Autodesk Inventor part; units mm, degrees
(part 2 of 3)
  measures "d19" distance of L6.end L4.start
  measures "d20" distance between parallel lines of L1 L7
  measures "d21" distance of L0.start L1.end
  measures "d22" distance between parallel lines of L0 L4
extrude "Extrusion4" cut sketch "Sketch4" against normal blind 5.08 contours S0 L8 L9 S1 S2 S3 S4 S5 S6 S7 S8 L10 L11 S9 S10 S11 S12 S13 S14 S15 | S16 S17 L12 L13 L14 S18 S19 S20 S21 L15 L16 L17 S22 S23 | S24 S25 L18 L19 L20 S26 S27 S28 L21 S29 | L28 L29 L30 L31 | S38 S39 L32 L33 L34 S40 S41 S42 L35 S43 | L42 L43 L44 L45 L46 L47 L48 L49 | S52 L53 L54 S53 S54 S55 S56 S57 S58 S59 S60 L55 L56 S61 S62 S63 S64 S65 S66 S67 | L57 L58 L59 L60 L61 L62 L63 L64 L65 L66 L67 L68 | L69 L70 L71 L72 L73 L74 L75 L76 L77 L78 | S68 S69 S70 S71 S72 S73 S74 S75 | S82 S83 L79 L80 L81 S84 S85 S86 S87 L82 L83 L84 S88 S89 | L85 L86 L87 L88 L89 L90 L91 S90 S91 S92 L92 | L96 L97 L98 L99 L100 L101 L102 L103 L104 L105 L106 L107 | L108 L109 L110 L111 L112 L113 L114 L115 L116 L117 L118 L119 | L120 L121 L122 L123 L124 L125 L126 S97 S98 S99 L127 | L131 L132 L133 L134 L135 L136 L137 L138 | L139 L150 L146 | L146 L150 L151 L152 L153 L154 L155 L156 L157 | L139 L140 L141 L142 L143 L144 L145 S104 S105 S106 L146 L150 | L161 L162 L163 L164 L165 L166 L167 L168 L169 L170 | S111 L171 L172 S112 S113 S114 S115 S116 S117 S118 S119 L173 L174 S120 S121 S122 S123 S124 S125 S126 | L175 L176 L177 L178 L179 L180 L181 L182 L183 L184 | S127 S128 S129 S130 S131 S132 S133 S134 | L185 L186 L187 L188 L189 L190 L191 S141 S142 S143 L192 | L196 L197 L198 L199 L200 L201 L202 L203 L204 L205 L206 L207 L208
sketch "Sketch5" plane through (0, -25.4, 0) normal (0, -1, 0) x (1, 0, 0)
  line L0 (0, 0) -> (203.2, 0) projected
  line L1 (203.2, 50.8) -> (0, 50.8) projected
  line L2 (0, 50.8) -> (0, 0) projected
  line L3 (203.2, 0) -> (203.2, 50.8) projected
  line L4 (8.4667, 48.26) -> (110.0667, 48.26) construction
  line L5 (110.0667, 48.26) -> (110.0667, 2.54) construction
  line L6 (110.0667, 2.54) -> (8.4667, 2.54) construction
  line L7 (8.4667, 2.54) -> (8.4667, 48.26) construction
  line L8 (118.5333, 38.1) -> (194.7333, 38.1) construction
  line L9 (194.7333, 38.1) -> (194.7333, 12.7) construction
  line L10 (194.7333, 12.7) -> (118.5333, 12.7) construction
  line L11 (118.5333, 12.7) -> (118.5333, 38.1) construction
  spline S0 degree 2 poles (23.465, 39.4772) (23.465, 38.2768) (21.9978, 36.9726) (20.7603, 36.9726) knots 0 0 0 1 2 2 2
  spline S1 degree 2 poles (20.7603, 36.9726) (20.4639, 36.9726) (19.4784, 37.0764) (19.145, 37.1505) knots 0 0 0 1 2 2 2
  line L12 (19.145, 37.1505) -> (19.145, 38.3213)
  line L13 (19.145, 38.3213) -> (19.2116, 38.3213)
  spline S2 degree 2 poles (19.2116, 38.3213) (19.4636, 38.2323) (20.212, 38.0249) (20.5973, 38.0249) knots 0 0 0 1 2 2 2
  spline S3 degree 2 poles (20.5973, 38.0249) (21.1605, 38.0249) (21.8348, 38.2842) (21.9904, 38.5213) knots 0 0 0 1 2 2 2
  spline S4 degree 2 poles (21.9904, 38.5213) (22.1608, 38.7659) (22.2498, 39.4772) (22.2498, 39.9441) knots 0 0 0 1 2 2 2
  line L14 (22.2498, 39.9441) -> (22.2498, 45.2719)
  line L15 (22.2498, 45.2719) -> (20.3157, 45.2719)
  line L16 (20.3157, 45.2719) -> (20.3157, 46.2426)
  line L17 (20.3157, 46.2426) -> (23.465, 46.2426)
  line L18 (23.465, 46.2426) -> (23.465, 39.4772)
  spline S5 degree 2 poles (28.452, 36.9059) (27.6443, 36.9059) (26.4439, 37.3283) (26.0215, 37.7507) knots 0 0 0 1 2 2 2
  spline S6 degree 2 poles (26.0215, 37.7507) (25.5398, 38.2249) (25.1471, 39.5587) (25.1471, 40.5369) knots 0 0 0 1 2 2 2
  line L19 (25.1471, 40.5369) -> (25.1471, 46.2426)
  line L20 (25.1471, 46.2426) -> (26.3623, 46.2426)
  line L21 (26.3623, 46.2426) -> (26.3623, 40.5369)
  spline S7 degree 2 poles (26.3623, 40.5369) (26.3623, 39.8996) (26.5254, 39.04) (26.7551, 38.6918) knots 0 0 0 1 2 2 2
  spline S8 degree 2 poles (26.7551, 38.6918) (26.9996, 38.3213) (27.8444, 37.9433) (28.452, 37.9433) knots 0 0 0 1 2 2 2
  spline S9 degree 2 poles (28.452, 37.9433) (29.0226, 37.9433) (29.9118, 38.3213) (30.1563, 38.6918) knots 0 0 0 1 2 2 2
  spline S10 degree 2 poles (30.1563, 38.6918) (30.386, 39.04) (30.549, 39.8922) (30.549, 40.5072) knots 0 0 0 1 2 2 2
  line L22 (30.549, 40.5072) -> (30.549, 46.2426)
  line L23 (30.549, 46.2426) -> (31.7643, 46.2426)
  line L24 (31.7643, 46.2426) -> (31.7643, 40.5369)
  spline S11 degree 2 poles (31.7643, 40.5369) (31.7643, 39.581) (31.3789, 38.2175) (30.8899, 37.7507) knots 0 0 0 1 2 2 2
  spline S12 degree 2 poles (30.8899, 37.7507) (30.4527, 37.3209) (29.2967, 36.9059) (28.452, 36.9059) knots 0 0 0 1 2 2 2
  spline S13 degree 2 poles (36.0547, 36.9356) (35.0617, 36.9356) (33.6687, 37.3505) (33.0536, 37.6469) knots 0 0 0 1 2 2 2
  line L25 (33.0536, 37.6469) -> (33.0536, 39.1734)
  line L26 (33.0536, 39.1734) -> (33.1425, 39.1734)
  spline S14 degree 2 poles (33.1425, 39.1734) (33.7428, 38.6103) (35.2618, 37.9878) (35.9658, 37.9878) knots 0 0 0 1 2 2 2
  spline S15 degree 2 poles (35.9658, 37.9878) (36.9735, 37.9878) (38.0035, 38.8251) (38.0035, 39.5143) knots 0 0 0 1 2 2 2
  spline S16 degree 2 poles (38.0035, 39.5143) (38.0035, 40.0626) (37.4626, 40.7443) (36.8772, 40.9148) knots 0 0 0 1 2 2 2
  spline S17 degree 2 poles (36.8772, 40.9148) (36.4548, 41.0333) (35.7509, 41.1964) (35.2248, 41.3297) knots 0 0 0 1 2 2 2
  spline S18 degree 2 poles (35.2248, 41.3297) (34.7505, 41.4557) (34.0021, 41.8336) (33.7131, 42.1374) knots 0 0 0 1 2 2 2
  spline S19 degree 2 poles (33.7131, 42.1374) (33.4315, 42.4412) (33.1203, 43.2564) (33.1203, 43.7899) knots 0 0 0 1 2 2 2
  spline S20 degree 2 poles (33.1203, 43.7899) (33.1203, 44.9014) (34.8543, 46.4056) (36.1955, 46.4056) knots 0 0 0 1 2 2 2
  spline S21 degree 2 poles (36.1955, 46.4056) (36.9661, 46.4056) (38.3296, 46.1018) (38.915, 45.8128) knots 0 0 0 1 2 2 2
  line L27 (38.915, 45.8128) -> (38.915, 44.3605)
  line L28 (38.915, 44.3605) -> (38.826, 44.3605)
  spline S22 degree 2 poles (38.826, 44.3605) (38.3889, 44.7606) (37.0254, 45.3534) (36.277, 45.3534) knots 0 0 0 1 2 2 2
  spline S23 degree 2 poles (36.277, 45.3534) (35.4322, 45.3534) (34.3874, 44.5605) (34.3874, 43.9158) knots 0 0 0 1 2 2 2
  spline S24 degree 2 poles (34.3874, 43.9158) (34.3874, 43.3379) (35.0025, 42.6487) (35.5804, 42.4931) knots 0 0 0 1 2 2 2
  spline S25 degree 2 poles (35.5804, 42.4931) (35.9658, 42.3894) (37.0847, 42.1226) (37.4552, 42.0115) knots 0 0 0 1 2 2 2
  spline S26 degree 2 poles (37.4552, 42.0115) (38.3963, 41.7225) (39.2706, 40.5591) (39.2706, 39.7069) knots 0 0 0 1 2 2 2
  spline S27 degree 2 poles (39.2706, 39.7069) (39.2706, 39.166) (38.8335, 38.1286) (38.4407, 37.7655) knots 0 0 0 1 2 2 2
  spline S28 degree 2 poles (38.4407, 37.7655) (38.0035, 37.3654) (36.892, 36.9356) (36.0547, 36.9356) knots 0 0 0 1 2 2 2
  line L29 (42.6422, 37.0986) -> (42.6422, 45.1607)
  line L30 (42.6422, 45.1607) -> (39.5745, 45.1607)
  line L31 (39.5745, 45.1607) -> (39.5745, 46.2426)
  line L32 (39.5745, 46.2426) -> (46.9252, 46.2426)
  line L33 (46.9252, 46.2426) -> (46.9252, 45.1607)
  line L34 (46.9252, 45.1607) -> (43.8575, 45.1607)
  line L35 (43.8575, 45.1607) -> (43.8575, 37.0986)
  line L36 (43.8575, 37.0986) -> (42.6422, 37.0986)
  line L37 (51.0378, 37.0986) -> (47.4958, 37.0986)
  line L38 (47.4958, 37.0986) -> (47.4958, 38.0323)
  line L39 (47.4958, 38.0323) -> (48.6592, 38.0323)
  line L40 (48.6592, 38.0323) -> (48.6592, 45.3089)
  line L41 (48.6592, 45.3089) -> (47.4958, 45.3089)
  line L42 (47.4958, 45.3089) -> (47.4958, 46.2426)
  line L43 (47.4958, 46.2426) -> (51.0378, 46.2426)
  line L44 (51.0378, 46.2426) -> (51.0378, 45.3089)
  line L45 (51.0378, 45.3089) -> (49.8744, 45.3089)
  line L46 (49.8744, 45.3089) -> (49.8744, 38.0323)
  line L47 (49.8744, 38.0323) -> (51.0378, 38.0323)
  line L48 (51.0378, 38.0323) -> (51.0378, 37.0986)
  line L49 (59.0851, 37.0986) -> (57.7217, 37.0986)
  line L50 (57.7217, 37.0986) -> (53.6758, 44.9829)
  line L51 (53.6758, 44.9829) -> (53.6758, 37.0986)
  line L52 (53.6758, 37.0986) -> (52.542, 37.0986)
  line L53 (52.542, 37.0986) -> (52.542, 46.2426)
  line L54 (52.542, 46.2426) -> (54.2686, 46.2426)
  line L55 (54.2686, 46.2426) -> (57.9514, 39.003)
  line L56 (57.9514, 39.003) -> (57.9514, 46.2426)
  line L57 (57.9514, 46.2426) -> (59.0851, 46.2426)
  line L58 (59.0851, 46.2426) -> (59.0851, 37.0986)
  line L59 (63.8794, 37.0986) -> (66.962, 46.2426)
  line L60 (66.962, 46.2426) -> (68.4588, 46.2426)
  line L61 (68.4588, 46.2426) -> (71.5414, 37.0986)
  line L62 (71.5414, 37.0986) -> (70.2595, 37.0986)
  line L63 (70.2595, 37.0986) -> (69.4295, 39.6551)
  line L64 (69.4295, 39.6551) -> (65.9394, 39.6551)
  line L65 (65.9394, 39.6551) -> (65.1095, 37.0986)
  line L66 (65.1095, 37.0986) -> (63.8794, 37.0986)
  line L67 (69.0961, 40.6925) -> (67.6808, 44.9977)
  line L68 (67.6808, 44.9977) -> (66.2729, 40.6925)
  line L69 (66.2729, 40.6925) -> (69.0961, 40.6925)
  line L70 (77.7066, 37.0986) -> (72.4084, 37.0986)
  line L71 (72.4084, 37.0986) -> (72.4084, 46.2426)
  line L72 (72.4084, 46.2426) -> (73.6236, 46.2426)
  line L73 (73.6236, 46.2426) -> (73.6236, 38.1805)
  line L74 (73.6236, 38.1805) -> (77.7066, 38.1805)
  line L75 (77.7066, 38.1805) -> (77.7066, 37.0986)
  line L76 (83.9607, 37.0986) -> (78.6625, 37.0986)
  line L77 (78.6625, 37.0986) -> (78.6625, 46.2426)
  line L78 (78.6625, 46.2426) -> (79.8777, 46.2426)
  line L79 (79.8777, 46.2426) -> (79.8777, 38.1805)
  line L80 (79.8777, 38.1805) -> (83.9607, 38.1805)
  line L81 (83.9607, 38.1805) -> (83.9607, 37.0986)
  line L82 (84.9165, 37.0986) -> (84.9165, 46.2426)
  line L83 (84.9165, 46.2426) -> (90.6371, 46.2426)
  line L84 (90.6371, 46.2426) -> (90.6371, 45.1607)
  line L85 (90.6371, 45.1607) -> (86.1318, 45.1607)
  line L86 (86.1318, 45.1607) -> (86.1318, 42.6561)
  line L87 (86.1318, 42.6561) -> (90.3333, 42.6561)
  line L88 (90.3333, 42.6561) -> (90.3333, 41.5743)
  line L89 (90.3333, 41.5743) -> (86.1318, 41.5743)
  line L90 (86.1318, 41.5743) -> (86.1318, 38.1805)
  line L91 (86.1318, 38.1805) -> (90.6371, 38.1805)
  line L92 (90.6371, 38.1805) -> (90.6371, 37.0986)
  line L93 (90.6371, 37.0986) -> (84.9165, 37.0986)
  line L94 (98.514, 37.0986) -> (97.1505, 37.0986)
  line L95 (97.1505, 37.0986) -> (93.1047, 44.9829)
  line L96 (93.1047, 44.9829) -> (93.1047, 37.0986)
  line L97 (93.1047, 37.0986) -> (91.9709, 37.0986)
  line L98 (91.9709, 37.0986) -> (91.9709, 46.2426)
  line L99 (91.9709, 46.2426) -> (93.6975, 46.2426)
  line L100 (93.6975, 46.2426) -> (97.3802, 39.003)
  line L101 (97.3802, 39.003) -> (97.3802, 46.2426)
  line L102 (97.3802, 46.2426) -> (98.514, 46.2426)
  line L103 (98.514, 46.2426) -> (98.514, 37.0986)
  line L104 (27.9889, 22.0432) -> (31.0714, 31.1872)
  line L105 (31.0714, 31.1872) -> (32.5683, 31.1872)
  line L106 (32.5683, 31.1872) -> (35.6508, 22.0432)
  line L107 (35.6508, 22.0432) -> (34.3689, 22.0432)
  line L108 (34.3689, 22.0432) -> (33.539, 24.5997)
  line L109 (33.539, 24.5997) -> (30.0488, 24.5997)
  line L110 (30.0488, 24.5997) -> (29.2189, 22.0432)
  line L111 (29.2189, 22.0432) -> (27.9889, 22.0432)
  line L112 (33.2055, 25.6371) -> (31.7902, 29.9424)
  line L113 (31.7902, 29.9424) -> (30.3823, 25.6371)
  line L114 (30.3823, 25.6371) -> (33.2055, 25.6371)
  line L115 (41.4381, 22.0432) -> (36.9772, 22.0432)
  line L116 (36.9772, 22.0432) -> (36.9772, 22.9769)
  line L117 (36.9772, 22.9769) -> (38.6371, 22.9769)
  line L118 (38.6371, 22.9769) -> (38.6371, 29.105)
  line L119 (38.6371, 29.105) -> (36.9772, 29.105)
  line L120 (36.9772, 29.105) -> (36.9772, 29.9424)
  spline S29 degree 2 poles (36.9772, 29.9424) (37.9183, 29.9424) (38.8075, 30.4759) (38.8668, 31.2169) knots 0 0 0 1 2 2 2
  line L121 (38.8668, 31.2169) -> (39.8153, 31.2169)
  line L122 (39.8153, 31.2169) -> (39.8153, 22.9769)
  line L123 (39.8153, 22.9769) -> (41.4381, 22.9769)
  line L124 (41.4381, 22.9769) -> (41.4381, 22.0432)
  line L125 (49.0037, 25.1851) -> (47.9145, 25.1851)
  line L126 (47.9145, 25.1851) -> (47.9145, 22.0432)
  line L127 (47.9145, 22.0432) -> (46.7363, 22.0432)
  line L128 (46.7363, 22.0432) -> (46.7363, 25.1851)
  line L129 (46.7363, 25.1851) -> (42.6978, 25.1851)
  line L130 (42.6978, 25.1851) -> (42.6978, 26.4745)
  line L131 (42.6978, 26.4745) -> (46.7881, 31.1872)
  line L132 (46.7881, 31.1872) -> (47.9145, 31.1872)
  line L133 (47.9145, 31.1872) -> (47.9145, 26.1706)
  line L134 (47.9145, 26.1706) -> (49.0037, 26.1706)
  line L135 (49.0037, 26.1706) -> (49.0037, 25.1851)
  line L136 (46.7363, 26.1706) -> (46.7363, 29.7423)
  line L137 (46.7363, 29.7423) -> (43.6611, 26.1706)
  line L138 (43.6611, 26.1706) -> (46.7363, 26.1706)
  spline S30 degree 2 poles (55.5246, 24.948) (55.5246, 24.2885) (55.1022, 23.1622) (54.7169, 22.7472) knots 0 0 0 1 2 2 2
  spline S31 degree 2 poles (54.7169, 22.7472) (54.3316, 22.3322) (53.183, 21.8506) (52.4717, 21.8506) knots 0 0 0 1 2 2 2
  spline S32 degree 2 poles (52.4717, 21.8506) (51.8196, 21.8506) (50.545, 22.1396) (50.0782, 22.3693) knots 0 0 0 1 2 2 2
  line L139 (50.0782, 22.3693) -> (50.0782, 23.666)
  line L140 (50.0782, 23.666) -> (50.1671, 23.666)
  spline S33 degree 2 poles (50.1671, 23.666) (50.3079, 23.5623) (50.834, 23.2955) (51.1527, 23.177) knots 0 0 0 1 2 2 2
  spline S34 degree 2 poles (51.1527, 23.177) (51.5158, 23.051) (52.116, 22.9102) (52.4939, 22.9102) knots 0 0 0 1 2 2 2
  spline S35 degree 2 poles (52.4939, 22.9102) (52.8644, 22.9102) (53.5609, 23.177) (53.8129, 23.466) knots 0 0 0 1 2 2 2
  spline S36 degree 2 poles (53.8129, 23.466) (54.0426, 23.7401) (54.2797, 24.4663) (54.2797, 24.9554) knots 0 0 0 1 2 2 2
  spline S37 degree 2 poles (54.2797, 24.9554) (54.2797, 25.4445) (54.0129, 26.0669) (53.761, 26.2744) knots 0 0 0 1 2 2 2
  spline S38 degree 2 poles (53.761, 26.2744) (53.5016, 26.5041) (52.731, 26.6968) (52.2642, 26.6968) knots 0 0 0 1 2 2 2
  spline S39 degree 2 poles (52.2642, 26.6968) (51.7603, 26.6968) (50.7599, 26.5411) (50.4561, 26.4745) knots 0 0 0 1 2 2 2
  line L141 (50.4561, 26.4745) -> (50.4561, 31.1872)
  line L142 (50.4561, 31.1872) -> (55.4727, 31.1872)
  line L143 (55.4727, 31.1872) -> (55.4727, 30.1128)
  line L144 (55.4727, 30.1128) -> (51.6343, 30.1128)
  line L145 (51.6343, 30.1128) -> (51.6343, 27.6749)
  spline S40 degree 2 poles (51.6343, 27.6749) (51.8566, 27.7045) (52.2864, 27.7268) (52.4642, 27.7268) knots 0 0 0 1 2 2 2
  spline S41 degree 2 poles (52.4642, 27.7268) (53.1682, 27.7268) (54.1389, 27.497) (54.5835, 27.1562) knots 0 0 0 1 2 2 2
  spline S42 degree 2 poles (54.5835, 27.1562) (55.0355, 26.8153) (55.5246, 25.7779) (55.5246, 24.948) knots 0 0 0 1 2 2 2
  spline S43 degree 2 poles (62.6234, 25.0073) (62.6234, 24.3033) (62.1566, 23.1103) (61.7639, 22.7102) knots 0 0 0 1 2 2 2
  spline S44 degree 2 poles (61.7639, 22.7102) (61.3563, 22.2878) (60.3337, 21.8506) (59.7187, 21.8506) knots 0 0 0 1 2 2 2
  spline S45 degree 2 poles (59.7187, 21.8506) (59.1036, 21.8506) (58.0885, 22.2655) (57.7031, 22.6805) knots 0 0 0 1 2 2 2
  spline S46 degree 2 poles (57.7031, 22.6805) (57.2289, 23.177) (56.6954, 24.8442) (56.6954, 26.0595) knots 0 0 0 1 2 2 2
  spline S47 degree 2 poles (56.6954, 26.0595) (56.6954, 27.2525) (57.1844, 29.1717) (57.6957, 29.8831) knots 0 0 0 1 2 2 2
  spline S48 degree 2 poles (57.6957, 29.8831) (58.1922, 30.5796) (59.7631, 31.3577) (60.7931, 31.3577) knots 0 0 0 1 2 2 2
  spline S49 degree 2 poles (60.7931, 31.3577) (61.0969, 31.3577) (61.6305, 31.2984) (61.8305, 31.2317) knots 0 0 0 1 2 2 2
  line L146 (61.8305, 31.2317) -> (61.8305, 30.0535)
  line L147 (61.8305, 30.0535) -> (61.7787, 30.0535)
  spline S50 degree 2 poles (61.7787, 30.0535) (61.6082, 30.1424) (60.9858, 30.298) (60.6301, 30.298) knots 0 0 0 1 2 2 2
  spline S51 degree 2 poles (60.6301, 30.298) (59.489, 30.298) (58.0885, 28.7568) (57.9551, 27.2451) knots 0 0 0 1 2 2 2
  spline S52 degree 2 poles (57.9551, 27.2451) (58.3923, 27.5489) (59.3111, 27.8824) (59.8595, 27.8824) knots 0 0 0 1 2 2 2
  spline S53 degree 2 poles (59.8595, 27.8824) (60.393, 27.8824) (61.1933, 27.6675) (61.6305, 27.3414) knots 0 0 0 1 2 2 2
  spline S54 degree 2 poles (61.6305, 27.3414) (62.1344, 26.9635) (62.6234, 25.7927) (62.6234, 25.0073) knots 0 0 0 1 2 2 2
  spline S55 degree 2 poles (61.3785, 24.9554) (61.3785, 25.5186) (61.0821, 26.2818) (60.7561, 26.5486) knots 0 0 0 1 2 2 2
  spline S56 degree 2 poles (60.7561, 26.5486) (60.5116, 26.7412) (59.9039, 26.8672) (59.5853, 26.8672) knots 0 0 0 1 2 2 2
  spline S57 degree 2 poles (59.5853, 26.8672) (59.1555, 26.8672) (58.3478, 26.6078) (57.9551, 26.3633) knots 0 0 0 1 2 2 2
  spline S58 degree 2 poles (57.9551, 26.3633) (57.9477, 26.2299) (57.9329, 25.978) (57.9329, 25.7853) knots 0 0 0 1 2 2 2
  spline S59 degree 2 poles (57.9329, 25.7853) (57.9329, 24.8368) (58.3034, 23.6735) (58.5849, 23.3696) knots 0 0 0 1 2 2 2
  spline S60 degree 2 poles (58.5849, 23.3696) (58.8443, 23.0807) (59.4075, 22.8509) (59.7261, 22.8509) knots 0 0 0 1 2 2 2
  spline S61 degree 2 poles (59.7261, 22.8509) (60.4671, 22.8509) (61.3785, 23.9032) (61.3785, 24.9554) knots 0 0 0 1 2 2 2
  spline S62 degree 2 poles (69.4851, 25.0073) (69.4851, 24.3033) (69.0183, 23.1103) (68.6256, 22.7102) knots 0 0 0 1 2 2 2
  spline S63 degree 2 poles (68.6256, 22.7102) (68.218, 22.2878) (67.1954, 21.8506) (66.5804, 21.8506) knots 0 0 0 1 2 2 2
  spline S64 degree 2 poles (66.5804, 21.8506) (65.9654, 21.8506) (64.9502, 22.2655) (64.5649, 22.6805) knots 0 0 0 1 2 2 2
  spline S65 degree 2 poles (64.5649, 22.6805) (64.0906, 23.177) (63.5571, 24.8442) (63.5571, 26.0595) knots 0 0 0 1 2 2 2
  spline S66 degree 2 poles (63.5571, 26.0595) (63.5571, 27.2525) (64.0461, 29.1717) (64.5574, 29.8831) knots 0 0 0 1 2 2 2
  spline S67 degree 2 poles (64.5574, 29.8831) (65.0539, 30.5796) (66.6248, 31.3577) (67.6548, 31.3577) knots 0 0 0 1 2 2 2
  spline S68 degree 2 poles (67.6548, 31.3577) (67.9587, 31.3577) (68.4922, 31.2984) (68.6922, 31.2317) knots 0 0 0 1 2 2 2
  line L148 (68.6922, 31.2317) -> (68.6922, 30.0535)
  line L149 (68.6922, 30.0535) -> (68.6404, 30.0535)
  spline S69 degree 2 poles (68.6404, 30.0535) (68.4699, 30.1424) (67.8475, 30.298) (67.4918, 30.298) knots 0 0 0 1 2 2 2
  spline S70 degree 2 poles (67.4918, 30.298) (66.3507, 30.298) (64.9502, 28.7568) (64.8168, 27.2451) knots 0 0 0 1 2 2 2
  spline S71 degree 2 poles (64.8168, 27.2451) (65.254, 27.5489) (66.1728, 27.8824) (66.7212, 27.8824) knots 0 0 0 1 2 2 2
  spline S72 degree 2 poles (66.7212, 27.8824) (67.2547, 27.8824) (68.055, 27.6675) (68.4922, 27.3414) knots 0 0 0 1 2 2 2
  spline S73 degree 2 poles (68.4922, 27.3414) (68.9961, 26.9635) (69.4851, 25.7927) (69.4851, 25.0073) knots 0 0 0 1 2 2 2
  spline S74 degree 2 poles (68.2402, 24.9554) (68.2402, 25.5186) (67.9438, 26.2818) (67.6178, 26.5486) knots 0 0 0 1 2 2 2
  spline S75 degree 2 poles (67.6178, 26.5486) (67.3733, 26.7412) (66.7656, 26.8672) (66.447, 26.8672) knots 0 0 0 1 2 2 2
  spline S76 degree 2 poles (66.447, 26.8672) (66.0172, 26.8672) (65.2095, 26.6078) (64.8168, 26.3633) knots 0 0 0 1 2 2 2
  spline S77 degree 2 poles (64.8168, 26.3633) (64.8094, 26.2299) (64.7946, 25.978) (64.7946, 25.7853) knots 0 0 0 1 2 2 2
  spline S78 degree 2 poles (64.7946, 25.7853) (64.7946, 24.8368) (65.1651, 23.6735) (65.4466, 23.3696) knots 0 0 0 1 2 2 2
  spline S79 degree 2 poles (65.4466, 23.3696) (65.706, 23.0807) (66.2692, 22.8509) (66.5878, 22.8509) knots 0 0 0 1 2 2 2
  spline S80 degree 2 poles (66.5878, 22.8509) (67.3288, 22.8509) (68.2402, 23.9032) (68.2402, 24.9554) knots 0 0 0 1 2 2 2
  spline S81 degree 2 poles (76.2579, 26.6152) (76.2579, 24.1551) (74.8278, 21.8506) (73.3383, 21.8506) knots 0 0 0 1 2 2 2
  spline S82 degree 2 poles (73.3383, 21.8506) (71.8267, 21.8506) (70.4114, 24.1996) (70.4114, 26.6078) knots 0 0 0 1 2 2 2
  spline S83 degree 2 poles (70.4114, 26.6078) (70.4114, 29.0828) (71.8415, 31.3725) (73.3383, 31.3725) knots 0 0 0 1 2 2 2
  spline S84 degree 2 poles (73.3383, 31.3725) (74.8426, 31.3725) (76.2579, 29.0013) (76.2579, 26.6152) knots 0 0 0 1 2 2 2
  spline S85 degree 2 poles (74.687, 23.8291) (74.8648, 24.2811) (75.013, 25.6742) (75.013, 26.6152) knots 0 0 0 1 2 2 2
  spline S86 degree 2 poles (75.013, 26.6152) (75.013, 27.5563) (74.8648, 28.942) (74.6796, 29.4088) knots 0 0 0 1 2 2 2
  spline S87 degree 2 poles (74.6796, 29.4088) (74.4943, 29.8757) (73.8496, 30.3573) (73.3383, 30.3573) knots 0 0 0 1 2 2 2
  spline S88 degree 2 poles (73.3383, 30.3573) (72.8271, 30.3573) (72.1676, 29.8757) (71.9749, 29.394) knots 0 0 0 1 2 2 2
  spline S89 degree 2 poles (71.9749, 29.394) (71.7896, 28.9272) (71.6563, 27.5045) (71.6563, 26.6078) knots 0 0 0 1 2 2 2
  spline S90 degree 2 poles (71.6563, 26.6078) (71.6563, 25.6445) (71.7748, 24.3552) (71.9675, 23.8513) knots 0 0 0 1 2 2 2
  spline S91 degree 2 poles (71.9675, 23.8513) (72.1453, 23.3771) (72.8048, 22.8658) (73.3383, 22.8658) knots 0 0 0 1 2 2 2
  spline S92 degree 2 poles (73.3383, 22.8658) (73.8422, 22.8658) (74.5017, 23.3474) (74.687, 23.8291) knots 0 0 0 1 2 2 2
  line L150 (83.1715, 29.8164) -> (79.2145, 22.0432)
  line L151 (79.2145, 22.0432) -> (77.9103, 22.0432)
  line L152 (77.9103, 22.0432) -> (82.0896, 30.1128)
  line L153 (82.0896, 30.1128) -> (77.3694, 30.1128)
  line L154 (77.3694, 30.1128) -> (77.3694, 31.1872)
  line L155 (77.3694, 31.1872) -> (83.1715, 31.1872)
  line L156 (83.1715, 31.1872) -> (83.1715, 29.8164)
  line L157 (89.47, 22.0432) -> (85.0092, 22.0432)
  line L158 (85.0092, 22.0432) -> (85.0092, 22.9769)
  line L159 (85.0092, 22.9769) -> (86.669, 22.9769)
  line L160 (86.669, 22.9769) -> (86.669, 29.105)
  line L161 (86.669, 29.105) -> (85.0092, 29.105)
  line L162 (85.0092, 29.105) -> (85.0092, 29.9424)
  spline S93 degree 2 poles (85.0092, 29.9424) (85.9503, 29.9424) (86.8395, 30.4759) (86.8987, 31.2169) knots 0 0 0 1 2 2 2
  line L163 (86.8987, 31.2169) -> (87.8472, 31.2169)
  line L164 (87.8472, 31.2169) -> (87.8472, 22.9769)
  line L165 (87.8472, 22.9769) -> (89.47, 22.9769)
  line L166 (89.47, 22.9769) -> (89.47, 22.0432)
  spline S94 degree 2 poles (13.1391, 6.7952) (13.1391, 5.6244) (11.8794, 4.3944) (10.7753, 4.3944) knots 0 0 0 1 2 2 2
  spline S95 degree 2 poles (10.7753, 4.3944) (10.5827, 4.3944) (10.1084, 4.4314) (9.8787, 4.4685) knots 0 0 0 1 2 2 2
  line L167 (9.8787, 4.4685) -> (9.8787, 5.5059)
  line L168 (9.8787, 5.5059) -> (9.9454, 5.5059)
  spline S96 degree 2 poles (9.9454, 5.5059) (10.0788, 5.4762) (10.4048, 5.417) (10.553, 5.417) knots 0 0 0 1 2 2 2
  spline S97 degree 2 poles (10.553, 5.417) (11.0124, 5.417) (11.6126, 5.6467) (11.7534, 5.8912) knots 0 0 0 1 2 2 2
  spline S98 degree 2 poles (11.7534, 5.8912) (11.8942, 6.1135) (11.9831, 6.7878) (11.9831, 7.2695) knots 0 0 0 1 2 2 2
  line L169 (11.9831, 7.2695) -> (11.9831, 12.8937)
  line L170 (11.9831, 12.8937) -> (10.7457, 12.8937)
  line L171 (10.7457, 12.8937) -> (10.7457, 13.8496)
  line L172 (10.7457, 13.8496) -> (13.1391, 13.8496)
  line L173 (13.1391, 13.8496) -> (13.1391, 6.7952)
  line L174 (13.1465, 14.9907) -> (11.8349, 14.9907)
  line L175 (11.8349, 14.9907) -> (11.8349, 16.1912)
  line L176 (11.8349, 16.1912) -> (13.1465, 16.1912)
  line L177 (13.1465, 16.1912) -> (13.1465, 14.9907)
  spline S99 degree 2 poles (20.564, 10.5299) (20.564, 8.8478) (18.9338, 6.7952) (17.7037, 6.7952) knots 0 0 0 1 2 2 2
  spline S100 degree 2 poles (17.7037, 6.7952) (17.148, 6.7952) (16.3551, 7.0694) (15.9698, 7.3065) knots 0 0 0 1 2 2 2
  line L178 (15.9698, 7.3065) -> (15.8957, 6.9879)
  line L179 (15.8957, 6.9879) -> (14.8138, 6.9879)
  line L180 (14.8138, 6.9879) -> (14.8138, 16.5394)
  line L181 (14.8138, 16.5394) -> (15.9698, 16.5394)
  line L182 (15.9698, 16.5394) -> (15.9698, 13.1308)
  spline S101 degree 2 poles (15.9698, 13.1308) (16.4069, 13.5236) (17.4221, 14.0423) (18.0668, 14.0423) knots 0 0 0 1 2 2 2
  spline S102 degree 2 poles (18.0668, 14.0423) (19.2302, 14.0423) (20.564, 12.1823) (20.564, 10.5299) knots 0 0 0 1 2 2 2
  spline S103 degree 2 poles (19.371, 10.441) (19.371, 11.671) (18.6226, 12.9456) (17.7926, 12.9456) knots 0 0 0 1 2 2 2
  spline S104 degree 2 poles (17.7926, 12.9456) (17.3258, 12.9456) (16.3625, 12.501) (15.9698, 12.1601) knots 0 0 0 1 2 2 2
  line L183 (15.9698, 12.1601) -> (15.9698, 8.2254)
  spline S105 degree 2 poles (15.9698, 8.2254) (16.4069, 8.0105) (17.0813, 7.8326) (17.4814, 7.8326) knots 0 0 0 1 2 2 2
  spline S106 degree 2 poles (17.4814, 7.8326) (18.3632, 7.8326) (19.371, 9.0849) (19.371, 10.441) knots 0 0 0 1 2 2 2
  spline S107 degree 2 poles (25.588, 7.7141) (25.4472, 7.6103) (24.973, 7.2398) (24.7507, 7.1287) knots 0 0 0 1 2 2 2
  spline S108 degree 2 poles (24.7507, 7.1287) (24.4469, 6.9657) (23.8763, 6.7952) (23.3576, 6.7952) knots 0 0 0 1 2 2 2
  spline S109 degree 2 poles (23.3576, 6.7952) (22.9352, 6.7952) (22.172, 7.1139) (21.883, 7.4029) knots 0 0 0 1 2 2 2
  spline S110 degree 2 poles (21.883, 7.4029) (21.6088, 7.6844) (21.2754, 8.5144) (21.2754, 8.9738) knots 0 0 0 1 2 2 2
  spline S111 degree 2 poles (21.2754, 8.9738) (21.2754, 9.6852) (21.8756, 10.6929) (22.5276, 10.9819) knots 0 0 0 1 2 2 2
  spline S112 degree 2 poles (22.5276, 10.9819) (23.1056, 11.2487) (24.6766, 11.4487) (25.588, 11.5006) knots 0 0 0 1 2 2 2
  line L184 (25.588, 11.5006) -> (25.588, 11.7229)
  spline S113 degree 2 poles (25.588, 11.7229) (25.588, 12.1231) (25.3435, 12.6195) (25.1212, 12.7603) knots 0 0 0 1 2 2 2
  spline S114 degree 2 poles (25.1212, 12.7603) (24.8989, 12.9011) (24.2616, 12.99) (23.9207, 12.99) knots 0 0 0 1 2 2 2
  spline S115 degree 2 poles (23.9207, 12.99) (23.5206, 12.99) (22.4387, 12.7529) (21.8978, 12.5232) knots 0 0 0 1 2 2 2
  line L185 (21.8978, 12.5232) -> (21.8311, 12.5232)
  line L186 (21.8311, 12.5232) -> (21.8311, 13.7014)
  spline S116 degree 2 poles (21.8311, 13.7014) (22.1497, 13.7903) (23.3428, 14.0126) (23.9281, 14.0126) knots 0 0 0 1 2 2 2
  spline S117 degree 2 poles (23.9281, 14.0126) (24.6395, 14.0126) (25.6102, 13.7903) (25.9956, 13.5013) knots 0 0 0 1 2 2 2
  spline S118 degree 2 poles (25.9956, 13.5013) (26.3735, 13.2197) (26.744, 12.3231) (26.744, 11.6785) knots 0 0 0 1 2 2 2
  line L187 (26.744, 11.6785) -> (26.744, 6.9879)
  line L188 (26.744, 6.9879) -> (25.588, 6.9879)
  line L189 (25.588, 6.9879) -> (25.588, 7.7141)
  line L190 (25.588, 8.6774) -> (25.588, 10.5818)
  spline S119 degree 2 poles (25.588, 10.5818) (25.173, 10.5447) (23.9207, 10.4187) (23.528, 10.3002) knots 0 0 0 1 2 2 2
  spline S120 degree 2 poles (23.528, 10.3002) (23.0686, 10.1594) (22.4684, 9.574) (22.4684, 9.0553) knots 0 0 0 1 2 2 2
  spline S121 degree 2 poles (22.4684, 9.0553) (22.4684, 8.4625) (23.1353, 7.8623) (23.7725, 7.8623) knots 0 0 0 1 2 2 2
  spline S122 degree 2 poles (23.7725, 7.8623) (24.3135, 7.8623) (25.2027, 8.3291) (25.588, 8.6774) knots 0 0 0 1 2 2 2
  line L191 (29.545, 6.9879) -> (28.389, 6.9879)
  line L192 (28.389, 6.9879) -> (28.389, 16.5394)
  line L193 (28.389, 16.5394) -> (29.545, 16.5394)
  line L194 (29.545, 16.5394) -> (29.545, 6.9879)
  line L195 (32.4201, 6.9879) -> (31.2641, 6.9879)
  line L196 (31.2641, 6.9879) -> (31.2641, 16.5394)
  line L197 (31.2641, 16.5394) -> (32.4201, 16.5394)
  line L198 (32.4201, 16.5394) -> (32.4201, 6.9879)
  spline S123 degree 2 poles (37.0958, 6.8323) (35.4508, 6.8323) (33.6427, 8.6774) (33.6427, 10.3817) knots 0 0 0 1 2 2 2
  spline S124 degree 2 poles (33.6427, 10.3817) (33.6427, 12.0564) (35.3989, 14.0423) (36.8142, 14.0423) knots 0 0 0 1 2 2 2
  spline S125 degree 2 poles (36.8142, 14.0423) (37.4515, 14.0423) (38.437, 13.6718) (38.8001, 13.279) knots 0 0 0 1 2 2 2
  spline S126 degree 2 poles (38.8001, 13.279) (39.1706, 12.8863) (39.5633, 11.7526) (39.5633, 10.93) knots 0 0 0 1 2 2 2
  line L199 (39.5633, 10.93) -> (39.5633, 10.3002)
  line L200 (39.5633, 10.3002) -> (34.8135, 10.3002)
  spline S127 degree 2 poles (34.8135, 10.3002) (34.8135, 9.1072) (36.0139, 7.84) (37.081, 7.84) knots 0 0 0 1 2 2 2
  spline S128 degree 2 poles (37.081, 7.84) (37.4589, 7.84) (38.1925, 8.0105) (38.4889, 8.1439) knots 0 0 0 1 2 2 2
  spline S129 degree 2 poles (38.4889, 8.1439) (38.8001, 8.2921) (39.2299, 8.5514) (39.3707, 8.67) knots 0 0 0 1 2 2 2
  line L201 (39.3707, 8.67) -> (39.4374, 8.67)
  line L202 (39.4374, 8.67) -> (39.4374, 7.4103)
  spline S130 degree 2 poles (39.4374, 7.4103) (39.2373, 7.3288) (38.6297, 7.0916) (38.3926, 7.0249) knots 0 0 0 1 2 2 2
  spline S131 degree 2 poles (38.3926, 7.0249) (38.0591, 6.9286) (37.5108, 6.8323) (37.0958, 6.8323) knots 0 0 0 1 2 2 2
  spline S132 degree 2 poles (38.437, 11.182) (38.4222, 11.6488) (38.2295, 12.3305) (38.0443, 12.5602) knots 0 0 0 1 2 2 2
  spline S133 degree 2 poles (38.0443, 12.5602) (37.8442, 12.8196) (37.2144, 13.0938) (36.7475, 13.0938) knots 0 0 0 1 2 2 2
  spline S134 degree 2 poles (36.7475, 13.0938) (36.2881, 13.0938) (35.6434, 12.8196) (35.3767, 12.5528) knots 0 0 0 1 2 2 2
  spline S135 degree 2 poles (35.3767, 12.5528) (35.1173, 12.2787) (34.8506, 11.6192) (34.8135, 11.182) knots 0 0 0 1 2 2 2
  line L203 (34.8135, 11.182) -> (38.437, 11.182)
  line L204 (46.1212, 6.9879) -> (44.9653, 6.9879)
  line L205 (44.9653, 6.9879) -> (44.9653, 10.9004)
  spline S136 degree 2 poles (44.9653, 10.9004) (44.9653, 11.3746) (44.8764, 12.1897) (44.743, 12.4343) knots 0 0 0 1 2 2 2
  spline S137 degree 2 poles (44.743, 12.4343) (44.6022, 12.6936) (44.0983, 12.9456) (43.6685, 12.9456) knots 0 0 0 1 2 2 2
  spline S138 degree 2 poles (43.6685, 12.9456) (43.2387, 12.9456) (42.3273, 12.4861) (41.8901, 12.1156) knots 0 0 0 1 2 2 2
  line L206 (41.8901, 12.1156) -> (41.8901, 6.9879)
  line L207 (41.8901, 6.9879) -> (40.7341, 6.9879)
  line L208 (40.7341, 6.9879) -> (40.7341, 13.8496)
  line L209 (40.7341, 13.8496) -> (41.8901, 13.8496)
  line L210 (41.8901, 13.8496) -> (41.8901, 13.0864)
  spline S139 degree 2 poles (41.8901, 13.0864) (42.4088, 13.5532) (43.4092, 14.0423) (43.9723, 14.0423) knots 0 0 0 1 2 2 2
  spline S140 degree 2 poles (43.9723, 14.0423) (44.9801, 14.0423) (46.1212, 12.7085) (46.1212, 11.4413) knots 0 0 0 1 2 2 2
  line L211 (46.1212, 11.4413) -> (46.1212, 6.9879)
  spline S141 degree 2 poles (57.5846, 11.0634) (57.5846, 10.2113) (57.1178, 8.6181) (56.6806, 7.9586) knots 0 0 0 1 2 2 2
  line L212 (56.6806, 7.9586) -> (54.1019, 7.9586)
  line L213 (54.1019, 7.9586) -> (53.9463, 8.67)
  spline S142 degree 2 poles (53.9463, 8.67) (53.5313, 8.3217) (52.8422, 7.9067) (52.2419, 7.9067) knots 0 0 0 1 2 2 2
  spline S143 degree 2 poles (52.2419, 7.9067) (51.3009, 7.9067) (50.093, 9.4258) (50.093, 10.8633) knots 0 0 0 1 2 2 2
  spline S144 degree 2 poles (50.093, 10.8633) (50.093, 12.3083) (51.575, 13.9163) (52.5309, 13.9163) knots 0 0 0 1 2 2 2
  spline S145 degree 2 poles (52.5309, 13.9163) (52.9755, 13.9163) (53.6128, 13.694) (53.9388, 13.5087) knots 0 0 0 1 2 2 2
  line L214 (53.9388, 13.5087) -> (53.9388, 13.8051)
  line L215 (53.9388, 13.8051) -> (54.9096, 13.8051)
  line L216 (54.9096, 13.8051) -> (54.9096, 8.6403)
  line L217 (54.9096, 8.6403) -> (56.3026, 8.6403)
  spline S146 degree 2 poles (56.3026, 8.6403) (56.5398, 9.0775) (56.7398, 10.4632) (56.7398, 11.0264) knots 0 0 0 1 2 2 2
  spline S147 degree 2 poles (56.7398, 11.0264) (56.7398, 13.0345) (54.6947, 15.4798) (52.7755, 15.4798) knots 0 0 0 1 2 2 2
  spline S148 degree 2 poles (52.7755, 15.4798) (50.96, 15.4798) (48.5962, 12.8344) (48.5962, 10.9449) knots 0 0 0 1 2 2 2
  spline S149 degree 2 poles (48.5962, 10.9449) (48.5962, 8.9219) (50.8933, 6.4099) (52.7458, 6.4099) knots 0 0 0 1 2 2 2
  spline S150 degree 2 poles (52.7458, 6.4099) (53.2423, 6.4099) (54.3464, 6.5433) (54.8355, 6.6915) knots 0 0 0 1 2 2 2
  line L218 (54.8355, 6.6915) -> (54.8355, 5.8245)
  spline S151 degree 2 poles (54.8355, 5.8245) (54.3168, 5.6985) (53.2571, 5.6022) (52.7384, 5.6022) knots 0 0 0 1 2 2 2
  spline S152 degree 2 poles (52.7384, 5.6022) (50.5673, 5.6022) (47.7144, 8.5885) (47.7144, 10.9597) knots 0 0 0 1 2 2 2
  spline S153 degree 2 poles (47.7144, 10.9597) (47.7144, 13.2123) (50.6562, 16.3097) (52.7681, 16.3097) knots 0 0 0 1 2 2 2
  spline S154 degree 2 poles (52.7681, 16.3097) (55.0281, 16.3097) (57.5846, 13.3976) (57.5846, 11.0634) knots 0 0 0 1 2 2 2
  line L219 (53.924, 9.4925) -> (53.924, 12.6714)
  spline S155 degree 2 poles (53.924, 12.6714) (53.5832, 12.8492) (53.0052, 13.0049) (52.6865, 13.0049) knots 0 0 0 1 2 2 2
  spline S156 degree 2 poles (52.6865, 13.0049) (51.99, 13.0049) (51.1453, 11.9674) (51.1453, 10.8782) knots 0 0 0 1 2 2 2
  spline S157 degree 2 poles (51.1453, 10.8782) (51.1453, 9.9) (51.7825, 8.8552) (52.4865, 8.8552) knots 0 0 0 1 2 2 2
  spline S158 degree 2 poles (52.4865, 8.8552) (52.857, 8.8552) (53.5906, 9.2109) (53.924, 9.4925) knots 0 0 0 1 2 2 2
  line L220 (64.513, 6.9879) -> (63.357, 6.9879)
  line L221 (63.357, 6.9879) -> (63.357, 7.7437)
  spline S159 degree 2 poles (63.357, 7.7437) (62.8235, 7.2769) (61.8676, 6.7952) (61.2748, 6.7952) knots 0 0 0 1 2 2 2
  spline S160 degree 2 poles (61.2748, 6.7952) (60.8302, 6.7952) (60.0373, 7.0916) (59.7483, 7.4103) knots 0 0 0 1 2 2 2
  spline S161 degree 2 poles (59.7483, 7.4103) (59.4519, 7.7289) (59.1259, 8.6996) (59.1259, 9.3962) knots 0 0 0 1 2 2 2
  line L222 (59.1259, 9.3962) -> (59.1259, 13.8496)
  line L223 (59.1259, 13.8496) -> (60.2818, 13.8496)
  line L224 (60.2818, 13.8496) -> (60.2818, 9.9371)
  spline S162 degree 2 poles (60.2818, 9.9371) (60.2818, 9.3887) (60.3634, 8.67) (60.5041, 8.4032) knots 0 0 0 1 2 2 2
  spline S163 degree 2 poles (60.5041, 8.4032) (60.6449, 8.1365) (61.1266, 7.8919) (61.5786, 7.8919) knots 0 0 0 1 2 2 2
  spline S164 degree 2 poles (61.5786, 7.8919) (62.001, 7.8919) (62.9569, 8.3736) (63.357, 8.7218) knots 0 0 0 1 2 2 2
  line L225 (63.357, 8.7218) -> (63.357, 13.8496)
  line L226 (63.357, 13.8496) -> (64.513, 13.8496)
  line L227 (64.513, 13.8496) -> (64.513, 6.9879)
  spline S165 degree 2 poles (68.9146, 6.8323) (68.2032, 6.8323) (67.025, 7.2695) (66.6026, 7.7141) knots 0 0 0 1 2 2 2
  spline S166 degree 2 poles (66.6026, 7.7141) (66.1802, 8.1513) (65.7134, 9.4999) (65.7134, 10.4039) knots 0 0 0 1 2 2 2
  spline S167 degree 2 poles (65.7134, 10.4039) (65.7134, 11.308) (66.1951, 12.6269) (66.6026, 13.0715) knots 0 0 0 1 2 2 2
  spline S168 degree 2 poles (66.6026, 13.0715) (67.0102, 13.5236) (68.218, 14.0052) (68.9146, 14.0052) knots 0 0 0 1 2 2 2
  spline S169 degree 2 poles (68.9146, 14.0052) (69.4777, 14.0052) (70.5299, 13.6866) (70.9375, 13.4791) knots 0 0 0 1 2 2 2
  line L228 (70.9375, 13.4791) -> (70.9375, 12.1823)
  line L229 (70.9375, 12.1823) -> (70.8708, 12.1823)
  spline S170 degree 2 poles (70.8708, 12.1823) (70.7448, 12.2861) (70.3595, 12.5528) (70.0853, 12.6936) knots 0 0 0 1 2 2 2
  spline S171 degree 2 poles (70.0853, 12.6936) (69.8408, 12.8122) (69.1887, 12.9974) (68.8923, 12.9974) knots 0 0 0 1 2 2 2
  spline S172 degree 2 poles (68.8923, 12.9974) (67.9957, 12.9974) (66.9064, 11.6414) (66.9064, 10.4039) knots 0 0 0 1 2 2 2
  spline S173 degree 2 poles (66.9064, 10.4039) (66.9064, 9.1961) (67.9587, 7.84) (68.8923, 7.84) knots 0 0 0 1 2 2 2
  spline S174 degree 2 poles (68.8923, 7.84) (69.4555, 7.84) (70.4781, 8.3069) (70.8708, 8.67) knots 0 0 0 1 2 2 2
  line L230 (70.8708, 8.67) -> (70.9375, 8.67)
  line L231 (70.9375, 8.67) -> (70.9375, 7.3732)
  spline S175 degree 2 poles (70.9375, 7.3732) (70.7671, 7.2917) (70.2484, 7.062) (70.0409, 7.0101) knots 0 0 0 1 2 2 2
  spline S176 degree 2 poles (70.0409, 7.0101) (69.7445, 6.9212) (69.2776, 6.8323) (68.9146, 6.8323) knots 0 0 0 1 2 2 2
  spline S177 degree 2 poles (73.8422, 6.8249) (73.1531, 6.8249) (71.9601, 7.1954) (71.5673, 7.4029) knots 0 0 0 1 2 2 2
  line L232 (71.5673, 7.4029) -> (71.5673, 8.6996)
  line L233 (71.5673, 8.6996) -> (71.6266, 8.6996)
  spline S178 degree 2 poles (71.6266, 8.6996) (71.7748, 8.5811) (72.175, 8.2995) (72.5084, 8.1439) knots 0 0 0 1 2 2 2
  spline S179 degree 2 poles (72.5084, 8.1439) (72.7974, 8.0031) (73.5088, 7.7956) (73.8867, 7.7956) knots 0 0 0 1 2 2 2
  spline S180 degree 2 poles (73.8867, 7.7956) (74.1609, 7.7956) (74.7907, 7.9216) (74.9389, 8.0253) knots 0 0 0 1 2 2 2
  spline S181 degree 2 poles (74.9389, 8.0253) (75.1538, 8.1661) (75.3465, 8.4847) (75.3465, 8.8108) knots 0 0 0 1 2 2 2
  spline S182 degree 2 poles (75.3465, 8.8108) (75.3465, 9.2183) (74.9019, 9.6407) (74.3313, 9.7815) knots 0 0 0 1 2 2 2
  spline S183 degree 2 poles (74.3313, 9.7815) (74.109, 9.8334) (73.3976, 9.9816) (73.0938, 10.0631) knots 0 0 0 1 2 2 2
  spline S184 degree 2 poles (73.0938, 10.0631) (72.3084, 10.2928) (71.597, 11.2413) (71.597, 11.9156) knots 0 0 0 1 2 2 2
  spline S185 degree 2 poles (71.597, 11.9156) (71.597, 12.8492) (72.9975, 14.0126) (74.1535, 14.0126) knots 0 0 0 1 2 2 2
  spline S186 degree 2 poles (74.1535, 14.0126) (74.724, 14.0126) (75.88, 13.731) (76.2727, 13.5161) knots 0 0 0 1 2 2 2
  line L234 (76.2727, 13.5161) -> (76.2727, 12.2787)
  line L235 (76.2727, 12.2787) -> (76.2134, 12.2787)
  spline S187 degree 2 poles (76.2134, 12.2787) (75.7688, 12.6343) (74.687, 13.0419) (74.1312, 13.0419) knots 0 0 0 1 2 2 2
  spline S188 degree 2 poles (74.1312, 13.0419) (73.5607, 13.0419) (72.7752, 12.5602) (72.7752, 12.0786) knots 0 0 0 1 2 2 2
  spline S189 degree 2 poles (72.7752, 12.0786) (72.7752, 11.6414) (73.242, 11.219) (73.7607, 11.0856) knots 0 0 0 1 2 2 2
  spline S190 degree 2 poles (73.7607, 11.0856) (74.0127, 11.019) (74.6499, 10.8856) (74.9982, 10.8041) knots 0 0 0 1 2 2 2
  spline S191 degree 2 poles (74.9982, 10.8041) (75.754, 10.6114) (76.5247, 9.7296) (76.5247, 8.9664) knots 0 0 0 1 2 2 2
  spline S192 degree 2 poles (76.5247, 8.9664) (76.5247, 8.5218) (76.1764, 7.7363) (75.8355, 7.4473) knots 0 0 0 1 2 2 2
  spline S193 degree 2 poles (75.8355, 7.4473) (75.4724, 7.1435) (74.5462, 6.8249) (73.8422, 6.8249) knots 0 0 0 1 2 2 2
  line L236 (82.8751, 6.9879) -> (81.7191, 6.9879)
  line L237 (81.7191, 6.9879) -> (81.7191, 7.6844)
  spline S194 degree 2 poles (81.7191, 7.6844) (81.4524, 7.4621) (81.0596, 7.1657) (80.7929, 7.0398) knots 0 0 0 1 2 2 2
  spline S195 degree 2 poles (80.7929, 7.0398) (80.5483, 6.9212) (80.0222, 6.7952) (79.6739, 6.7952) knots 0 0 0 1 2 2 2
  spline S196 degree 2 poles (79.6739, 6.7952) (79.1108, 6.7952) (78.1623, 7.2621) (77.8288, 7.7141) knots 0 0 0 1 2 2 2
  spline S197 degree 2 poles (77.8288, 7.7141) (77.4954, 8.1661) (77.1249, 9.4999) (77.1249, 10.3669) knots 0 0 0 1 2 2 2
  spline S198 degree 2 poles (77.1249, 10.3669) (77.1249, 11.2709) (77.5917, 12.5899) (77.9993, 13.0864) knots 0 0 0 1 2 2 2
  spline S199 degree 2 poles (77.9993, 13.0864) (78.3772, 13.531) (79.4368, 14.0423) (80.0222, 14.0423) knots 0 0 0 1 2 2 2
  spline S200 degree 2 poles (80.0222, 14.0423) (80.5335, 14.0423) (81.2967, 13.8125) (81.7191, 13.5754) knots 0 0 0 1 2 2 2
  line L238 (81.7191, 13.5754) -> (81.7191, 16.5394)
  line L239 (81.7191, 16.5394) -> (82.8751, 16.5394)
  line L240 (82.8751, 16.5394) -> (82.8751, 6.9879)
  line L241 (81.7191, 8.6552) -> (81.7191, 12.6195)
  spline S201 degree 2 poles (81.7191, 12.6195) (81.2893, 12.827) (80.6076, 12.9826) (80.2149, 12.9826) knots 0 0 0 1 2 2 2
  spline S202 degree 2 poles (80.2149, 12.9826) (79.3257, 12.9826) (78.3179, 11.6488) (78.3179, 10.3891) knots 0 0 0 1 2 2 2
  spline S203 degree 2 poles (78.3179, 10.3891) (78.3179, 9.1739) (79.0885, 7.8919) (79.9407, 7.8919) knots 0 0 0 1 2 2 2
  spline S204 degree 2 poles (79.9407, 7.8919) (80.3927, 7.8919) (81.3116, 8.3069) (81.7191, 8.6552) knots 0 0 0 1 2 2 2
  line L242 (86.343, 6.9879) -> (84.8758, 6.9879)
  line L243 (84.8758, 6.9879) -> (84.8758, 8.7367)
  line L244 (84.8758, 8.7367) -> (86.343, 8.7367)
  line L245 (86.343, 8.7367) -> (86.343, 6.9879)
  spline S205 degree 2 poles (91.3374, 6.8323) (89.6923, 6.8323) (87.8843, 8.6774) (87.8843, 10.3817) knots 0 0 0 1 2 2 2
  spline S206 degree 2 poles (87.8843, 10.3817) (87.8843, 12.0564) (89.6405, 14.0423) (91.0558, 14.0423) knots 0 0 0 1 2 2 2
  spline S207 degree 2 poles (91.0558, 14.0423) (91.693, 14.0423) (92.6786, 13.6718) (93.0417, 13.279) knots 0 0 0 1 2 2 2
  spline S208 degree 2 poles (93.0417, 13.279) (93.4122, 12.8863) (93.8049, 11.7526) (93.8049, 10.93) knots 0 0 0 1 2 2 2
  line L246 (93.8049, 10.93) -> (93.8049, 10.3002)
  line L247 (93.8049, 10.3002) -> (89.0551, 10.3002)
  spline S209 degree 2 poles (89.0551, 10.3002) (89.0551, 9.1072) (90.2555, 7.84) (91.3225, 7.84) knots 0 0 0 1 2 2 2
  spline S210 degree 2 poles (91.3225, 7.84) (91.7005, 7.84) (92.434, 8.0105) (92.7304, 8.1439) knots 0 0 0 1 2 2 2
  spline S211 degree 2 poles (92.7304, 8.1439) (93.0417, 8.2921) (93.4715, 8.5514) (93.6122, 8.67) knots 0 0 0 1 2 2 2
  line L248 (93.6122, 8.67) -> (93.6789, 8.67)
  line L249 (93.6789, 8.67) -> (93.6789, 7.4103)
  spline S212 degree 2 poles (93.6789, 7.4103) (93.4789, 7.3288) (92.8712, 7.0916) (92.6341, 7.0249) knots 0 0 0 1 2 2 2
  spline S213 degree 2 poles (92.6341, 7.0249) (92.3007, 6.9286) (91.7523, 6.8323) (91.3374, 6.8323) knots 0 0 0 1 2 2 2
  spline S214 degree 2 poles (92.6786, 11.182) (92.6638, 11.6488) (92.4711, 12.3305) (92.2858, 12.5602) knots 0 0 0 1 2 2 2
  spline S215 degree 2 poles (92.2858, 12.5602) (92.0858, 12.8196) (91.4559, 13.0938) (90.9891, 13.0938) knots 0 0 0 1 2 2 2
  spline S216 degree 2 poles (90.9891, 13.0938) (90.5297, 13.0938) (89.885, 12.8196) (89.6182, 12.5528) knots 0 0 0 1 2 2 2
  spline S217 degree 2 poles (89.6182, 12.5528) (89.3589, 12.2787) (89.0921, 11.6192) (89.0551, 11.182) knots 0 0 0 1 2 2 2
  line L250 (89.0551, 11.182) -> (92.6786, 11.182)
  line L251 (100.2516, 6.9879) -> (99.0957, 6.9879)
  line L252 (99.0957, 6.9879) -> (99.0957, 7.6844)
  spline S218 degree 2 poles (99.0957, 7.6844) (98.8289, 7.4621) (98.4362, 7.1657) (98.1694, 7.0398) knots 0 0 0 1 2 2 2
  spline S219 degree 2 poles (98.1694, 7.0398) (97.9249, 6.9212) (97.3988, 6.7952) (97.0505, 6.7952) knots 0 0 0 1 2 2 2
  spline S220 degree 2 poles (97.0505, 6.7952) (96.4873, 6.7952) (95.5389, 7.2621) (95.2054, 7.7141) knots 0 0 0 1 2 2 2
  spline S221 degree 2 poles (95.2054, 7.7141) (94.872, 8.1661) (94.5014, 9.4999) (94.5014, 10.3669) knots 0 0 0 1 2 2 2
  spline S222 degree 2 poles (94.5014, 10.3669) (94.5014, 11.2709) (94.9683, 12.5899) (95.3758, 13.0864) knots 0 0 0 1 2 2 2
  spline S223 degree 2 poles (95.3758, 13.0864) (95.7537, 13.531) (96.8134, 14.0423) (97.3988, 14.0423) knots 0 0 0 1 2 2 2
  spline S224 degree 2 poles (97.3988, 14.0423) (97.9101, 14.0423) (98.6733, 13.8125) (99.0957, 13.5754) knots 0 0 0 1 2 2 2
  line L253 (99.0957, 13.5754) -> (99.0957, 16.5394)
  line L254 (99.0957, 16.5394) -> (100.2516, 16.5394)
  line L255 (100.2516, 16.5394) -> (100.2516, 6.9879)
  line L256 (99.0957, 8.6552) -> (99.0957, 12.6195)
  spline S225 degree 2 poles (99.0957, 12.6195) (98.6659, 12.827) (97.9842, 12.9826) (97.5914, 12.9826) knots 0 0 0 1 2 2 2
  spline S226 degree 2 poles (97.5914, 12.9826) (96.7022, 12.9826) (95.6945, 11.6488) (95.6945, 10.3891) knots 0 0 0 1 2 2 2
  spline S227 degree 2 poles (95.6945, 10.3891) (95.6945, 9.1739) (96.4651, 7.8919) (97.3173, 7.8919) knots 0 0 0 1 2 2 2
  spline S228 degree 2 poles (97.3173, 7.8919) (97.7693, 7.8919) (98.6881, 8.3069) (99.0957, 8.6552) knots 0 0 0 1 2 2 2
  line L257 (107.2616, 6.9879) -> (106.1056, 6.9879)
  line L258 (106.1056, 6.9879) -> (106.1056, 7.7437)
  spline S229 degree 2 poles (106.1056, 7.7437) (105.5721, 7.2769) (104.6162, 6.7952) (104.0234, 6.7952) knots 0 0 0 1 2 2 2
  spline S230 degree 2 poles (104.0234, 6.7952) (103.5788, 6.7952) (102.7859, 7.0916) (102.4969, 7.4103) knots 0 0 0 1 2 2 2
  spline S231 degree 2 poles (102.4969, 7.4103) (102.2005, 7.7289) (101.8744, 8.6996) (101.8744, 9.3962) knots 0 0 0 1 2 2 2
  line L259 (101.8744, 9.3962) -> (101.8744, 13.8496)
  line L260 (101.8744, 13.8496) -> (103.0304, 13.8496)
  line L261 (103.0304, 13.8496) -> (103.0304, 9.9371)
  spline S232 degree 2 poles (103.0304, 9.9371) (103.0304, 9.3887) (103.1119, 8.67) (103.2527, 8.4032) knots 0 0 0 1 2 2 2
  spline S233 degree 2 poles (103.2527, 8.4032) (103.3935, 8.1365) (103.8752, 7.8919) (104.3272, 7.8919) knots 0 0 0 1 2 2 2
  spline S234 degree 2 poles (104.3272, 7.8919) (104.7495, 7.8919) (105.7054, 8.3736) (106.1056, 8.7218) knots 0 0 0 1 2 2 2
  line L262 (106.1056, 8.7218) -> (106.1056, 13.8496)
  line L263 (106.1056, 13.8496) -> (107.2616, 13.8496)
  line L264 (107.2616, 13.8496) -> (107.2616, 6.9879)
  line L265 (143.7028, 28.3705) -> (142.4875, 28.3705)
  line L266 (142.4875, 28.3705) -> (142.4875, 36.2474)
  line L267 (142.4875, 36.2474) -> (140.1015, 30.8899)
  line L268 (140.1015, 30.8899) -> (139.3605, 30.8899)
  line L269 (139.3605, 30.8899) -> (136.9967, 36.2474)
  line L270 (136.9967, 36.2474) -> (136.9967, 28.3705)
  line L271 (136.9967, 28.3705) -> (135.863, 28.3705)
  line L272 (135.863, 28.3705) -> (135.863, 37.5145)
  line L273 (135.863, 37.5145) -> (137.5228, 37.5145)
  line L274 (137.5228, 37.5145) -> (139.8051, 32.4238)
  line L275 (139.8051, 32.4238) -> (142.0133, 37.5145)
  line L276 (142.0133, 37.5145) -> (143.7028, 37.5145)
  line L277 (143.7028, 37.5145) -> (143.7028, 28.3705)
  spline S235 degree 2 poles (148.749, 28.1778) (147.9413, 28.1778) (146.7409, 28.6002) (146.3185, 29.0226) knots 0 0 0 1 2 2 2
  spline S236 degree 2 poles (146.3185, 29.0226) (145.8369, 29.4968) (145.4442, 30.8306) (145.4442, 31.8088) knots 0 0 0 1 2 2 2
  line L278 (145.4442, 31.8088) -> (145.4442, 37.5145)
  line L279 (145.4442, 37.5145) -> (146.6594, 37.5145)
  line L280 (146.6594, 37.5145) -> (146.6594, 31.8088)
  spline S237 degree 2 poles (146.6594, 31.8088) (146.6594, 31.1715) (146.8224, 30.3119) (147.0521, 29.9637) knots 0 0 0 1 2 2 2
  spline S238 degree 2 poles (147.0521, 29.9637) (147.2967, 29.5932) (148.1414, 29.2152) (148.749, 29.2152) knots 0 0 0 1 2 2 2
  spline S239 degree 2 poles (148.749, 29.2152) (149.3196, 29.2152) (150.2088, 29.5932) (150.4534, 29.9637) knots 0 0 0 1 2 2 2
  spline S240 degree 2 poles (150.4534, 29.9637) (150.6831, 30.3119) (150.8461, 31.1641) (150.8461, 31.7791) knots 0 0 0 1 2 2 2
  line L281 (150.8461, 31.7791) -> (150.8461, 37.5145)
  line L282 (150.8461, 37.5145) -> (152.0613, 37.5145)
  line L283 (152.0613, 37.5145) -> (152.0613, 31.8088)
  spline S241 degree 2 poles (152.0613, 31.8088) (152.0613, 30.8529) (151.676, 29.4894) (151.1869, 29.0226) knots 0 0 0 1 2 2 2
  spline S242 degree 2 poles (151.1869, 29.0226) (150.7498, 28.5928) (149.5938, 28.1778) (148.749, 28.1778) knots 0 0 0 1 2 2 2
  spline S243 degree 2 poles (156.3517, 28.2075) (155.3588, 28.2075) (153.9657, 28.6224) (153.3507, 28.9188) knots 0 0 0 1 2 2 2
  line L284 (153.3507, 28.9188) -> (153.3507, 30.4453)
  line L285 (153.3507, 30.4453) -> (153.4396, 30.4453)
  spline S244 degree 2 poles (153.4396, 30.4453) (154.0398, 29.8821) (155.5589, 29.2597) (156.2628, 29.2597) knots 0 0 0 1 2 2 2
  spline S245 degree 2 poles (156.2628, 29.2597) (157.2706, 29.2597) (158.3006, 30.097) (158.3006, 30.7862) knots 0 0 0 1 2 2 2
  spline S246 degree 2 poles (158.3006, 30.7862) (158.3006, 31.3345) (157.7597, 32.0162) (157.1743, 32.1867) knots 0 0 0 1 2 2 2
  spline S247 degree 2 poles (157.1743, 32.1867) (156.7519, 32.3052) (156.0479, 32.4683) (155.5218, 32.6016) knots 0 0 0 1 2 2 2
  spline S248 degree 2 poles (155.5218, 32.6016) (155.0476, 32.7276) (154.2992, 33.1055) (154.0102, 33.4093) knots 0 0 0 1 2 2 2
  spline S249 degree 2 poles (154.0102, 33.4093) (153.7286, 33.7131) (153.4174, 34.5282) (153.4174, 35.0618) knots 0 0 0 1 2 2 2
  spline S250 degree 2 poles (153.4174, 35.0618) (153.4174, 36.1733) (155.1513, 37.6775) (156.4925, 37.6775) knots 0 0 0 1 2 2 2
  spline S251 degree 2 poles (156.4925, 37.6775) (157.2632, 37.6775) (158.6266, 37.3737) (159.212, 37.0847) knots 0 0 0 1 2 2 2
  line L286 (159.212, 37.0847) -> (159.212, 35.6323)
  line L287 (159.212, 35.6323) -> (159.1231, 35.6323)
  spline S252 degree 2 poles (159.1231, 35.6323) (158.6859, 36.0325) (157.3225, 36.6253) (156.5741, 36.6253) knots 0 0 0 1 2 2 2
  spline S253 degree 2 poles (156.5741, 36.6253) (155.7293, 36.6253) (154.6845, 35.8324) (154.6845, 35.1877) knots 0 0 0 1 2 2 2
  spline S254 degree 2 poles (154.6845, 35.1877) (154.6845, 34.6098) (155.2995, 33.9206) (155.8775, 33.765) knots 0 0 0 1 2 2 2
  spline S255 degree 2 poles (155.8775, 33.765) (156.2628, 33.6613) (157.3817, 33.3945) (157.7522, 33.2834) knots 0 0 0 1 2 2 2
  spline S256 degree 2 poles (157.7522, 33.2834) (158.6933, 32.9944) (159.5677, 31.831) (159.5677, 30.9788) knots 0 0 0 1 2 2 2
  spline S257 degree 2 poles (159.5677, 30.9788) (159.5677, 30.4379) (159.1305, 29.4005) (158.7378, 29.0374) knots 0 0 0 1 2 2 2
  spline S258 degree 2 poles (158.7378, 29.0374) (158.3006, 28.6373) (157.1891, 28.2075) (156.3517, 28.2075) knots 0 0 0 1 2 2 2
  line L288 (169.6528, 28.3705) -> (165.1919, 28.3705)
  line L289 (165.1919, 28.3705) -> (165.1919, 29.3042)
  line L290 (165.1919, 29.3042) -> (166.8518, 29.3042)
  line L291 (166.8518, 29.3042) -> (166.8518, 35.4323)
  line L292 (166.8518, 35.4323) -> (165.1919, 35.4323)
  line L293 (165.1919, 35.4323) -> (165.1919, 36.2696)
  spline S259 degree 2 poles (165.1919, 36.2696) (166.133, 36.2696) (167.0222, 36.8031) (167.0815, 37.5441) knots 0 0 0 1 2 2 2
  line L294 (167.0815, 37.5441) -> (168.03, 37.5441)
  line L295 (168.03, 37.5441) -> (168.03, 29.3042)
  line L296 (168.03, 29.3042) -> (169.6528, 29.3042)
  line L297 (169.6528, 29.3042) -> (169.6528, 28.3705)
  line L298 (170.6087, 28.3705) -> (173.6913, 37.5145)
  line L299 (173.6913, 37.5145) -> (175.1881, 37.5145)
  line L300 (175.1881, 37.5145) -> (178.2707, 28.3705)
  line L301 (178.2707, 28.3705) -> (176.9887, 28.3705)
  line L302 (176.9887, 28.3705) -> (176.1588, 30.927)
  line L303 (176.1588, 30.927) -> (172.6687, 30.927)
  line L304 (172.6687, 30.927) -> (171.8388, 28.3705)
  line L305 (171.8388, 28.3705) -> (170.6087, 28.3705)
  line L306 (175.8254, 31.9644) -> (174.41, 36.2696)
  line L307 (174.41, 36.2696) -> (173.0021, 31.9644)
  line L308 (173.0021, 31.9644) -> (175.8254, 31.9644)
  spline S260 degree 2 poles (122.1099, 13.1521) (121.117, 13.1521) (119.7239, 13.5671) (119.1088, 13.8635) knots 0 0 0 1 2 2 2